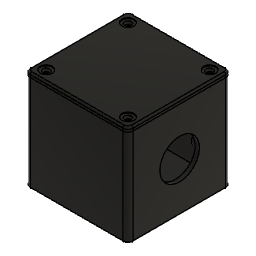
Transmitter_Box (Autodesk Fusion 360 design; units mm, degrees)
Autodesk Fusion 360 part; units mm, degrees
sketch "Sketch1" plane through (0, 0, 0) normal (0, 0, 1) x (1, 0, 0)
  line L0 (30, -30) -> (-30, -30)
  line L1 (-30, -30) -> (-30, 30)
  line L2 (-30, 30) -> (30, 30)
  line L3 (30, 30) -> (30, -30)
  line L4 (30, -30) -> (-30, 30) construction
  line L5 (-30, -30) -> (30, 30) construction
  dimension "d1" = 60
  dimension "d2" = 60
  constraint horizontal L0
  constraint perpendicular L0 L1
  constraint parallel L0 L2
  constraint parallel L1 L3
  constraint coincident L4 origin
  constraint coincident L5 origin
  measures "d1" distance of L1.end L2.end
  measures "d2" distance of L0.end L1.end
extrude "Extrude1" add sketch "Sketch1" along normal blind 2.4 makes body 1
sketch "Sketch2" plane through (0, 0, 2.4) normal (0, 0, 1) x (-1, 0, 0)
  line L0 (-30, -30) -> (30, -30)
  line L1 (30, -30) -> (30, 30)
  line L2 (30, 30) -> (-30, 30)
  line L3 (-30, 30) -> (-30, -30)
  line L4 (-27.6, -27.6) -> (27.6, -27.6)
  line L5 (27.6, -27.6) -> (27.6, 27.6)
  line L6 (27.6, 27.6) -> (-27.6, 27.6)
  line L7 (-27.6, 27.6) -> (-27.6, -27.6)
  line L8 (-27.6, -27.6) -> (27.6, 27.6) construction
  line L9 (27.6, -27.6) -> (-27.6, 27.6) construction
  dimension "d7" = 2.4
  dimension "d8" = 2.4
  constraint horizontal L4
  constraint perpendicular L4 L5
  constraint parallel L4 L6
  constraint parallel L5 L7
  constraint coincident L8 origin
  constraint coincident L9 origin
  measures "d7" distance of L0 L4
  measures "d8" distance of L1 L5
extrude "Extrude2" add sketch "Sketch2" along normal blind 54 bodies 1
sketch "Sketch3" plane through (0, 0, 56.4) normal (0, 0, 1) x (-1, 0, 0)
  line L0 (-27.6, -27.6) -> (-27.6, 27.6)
  line L1 (-27.6, 27.6) -> (27.6, 27.6)
  line L2 (27.6, 27.6) -> (27.6, -27.6)
  line L3 (27.6, -27.6) -> (-27.6, -27.6)
  line L4 (-30, 30) -> (-30, -30)
  line L5 (-30, -30) -> (30, -30)
  line L6 (30, -30) -> (30, 30)
  line L7 (30, 30) -> (-30, 30)
  line L8 (-30, 30) -> (30, 30)
  line L9 (30, 30) -> (30, -30)
  line L10 (30, -30) -> (-30, -30)
  line L11 (-30, -30) -> (-30, 30)
  constraint horizontal L8
  constraint vertical L9
  constraint horizontal L10
  constraint vertical L11
  constraint coincident L5.end L6.start
  constraint coincident L4.start L7.end
extrude "Extrude3" add sketch "Sketch3" along normal blind 2.4 separate body contours L0 L1 L2 L3 | L4 L5 L6 L7 L8 L9 L10 L11 makes body 2
sketch "Sketch4" plane through (-27.6, 0, 0) normal (1, 0, 0) x (0, 1, 0)
  line L0 (-27.6, 2.4) -> (27.6, 2.4)
  line L1 (27.6, 2.4) -> (27.6, 56.4)
  line L2 (27.6, 56.4) -> (-27.6, 56.4)
  line L3 (-27.6, 56.4) -> (-27.6, 2.4)
  line L4 (-27.6, 56.4) -> (-17.6, 56.4)
  line L5 (-17.6, 56.4) -> (-17.6, 52.4)
  line L6 (-17.6, 52.4) -> (-27.6, 52.4)
  line L7 (-27.6, 52.4) -> (-27.6, 56.4)
  line L8 (27.6, 56.4) -> (17.6, 56.4)
  line L9 (17.6, 56.4) -> (17.6, 52.4)
  line L10 (17.6, 52.4) -> (27.6, 52.4)
  line L11 (27.6, 52.4) -> (27.6, 56.4)
  dimension "d13" = 10
  dimension "d14" = 10
  dimension "d22" = 4
  dimension "d23" = 4
  constraint horizontal L4
  constraint vertical L5
  constraint horizontal L6
  constraint vertical L7
  constraint coincident L2.end L3.start
  constraint horizontal L8
  constraint vertical L9
  constraint horizontal L10
  constraint vertical L11
  constraint coincident L1.end L2.start
  measures "d13" distance of L5 L7
  measures "d14" distance of L9 L11
  measures "d22" distance of L4.end L5.end
  measures "d23" distance of L8.end L9.end
extrude "Extrude4" add sketch "Sketch4" along normal blind 10 contours L2 L3 L4 L5 L6 L7 | L1 L2 L8 L9 L10 L11 bodies 1
mirror "Mirror1" about plane through (0, 0, 0) normal (1, 0, 0) of "Extrude4"
sketch "Sketch8" plane through (0, 0, 56.4) normal (0, 0, 1) x (-1, 0, 0)
  line L0 (-27.6, -17.6) -> (-27.6, 17.6)
  line L1 (-27.6, 17.6) -> (-17.6, 17.6)
  line L2 (-17.6, 17.6) -> (-17.6, 27.6)
  line L3 (-17.6, 27.6) -> (17.6, 27.6)
  line L4 (17.6, 27.6) -> (17.6, 17.6)
  line L5 (17.6, 17.6) -> (27.6, 17.6)
  line L6 (27.6, 17.6) -> (27.6, -17.6)
  line L7 (27.6, -17.6) -> (17.6, -17.6)
  line L8 (17.6, -17.6) -> (17.6, -27.6)
  line L9 (17.6, -27.6) -> (-17.6, -27.6)
  line L10 (-17.6, -27.6) -> (-17.6, -17.6)
  line L11 (-17.6, -17.6) -> (-27.6, -17.6)
  line L12 (-30, 30) -> (-30, -30)
  line L13 (-30, -30) -> (30, -30)
  line L14 (30, -30) -> (30, 30)
  line L15 (30, 30) -> (-30, 30)
  circle A0 centre (-23.8, 23.8) radius 1.25
  circle A1 centre (23.8, 23.8) radius 1.25
  dimension "d27" = 2.5
  dimension "d28" = 6.2
  dimension "d29" = 6.2
  dimension "d30" = 2.5
  dimension "d31" = 6.2
  dimension "d32" = 6.2
  measures "d27" diameter of A0
  measures "d28" distance of L2 A0.centre
  measures "d29" distance of L1 A0.centre
  measures "d30" diameter of A1
  measures "d31" distance of L15 A1.centre
  measures "d32" distance of L14 A1.centre
extrude "Extrude5" cut sketch "Sketch8" against normal blind 4 contours A0 | A1 bodies 1
mirror "Mirror2" about plane through (0, 0, 0) normal (0, 1, 0) of "Extrude5"
sketch "Sketch9" plane through (0, 0, 58.8) normal (0, 0, 1) x (-1, 0, 0)
  line L0 (-30, -30) -> (30, -30)
  line L1 (30, -30) -> (30, 30)
  line L2 (30, 30) -> (-30, 30)
  line L3 (-30, 30) -> (-30, -30)
  circle A0 centre (-23.8, 23.8) radius 2
  circle A1 centre (23.8, 23.8) radius 2
  dimension "d37" = 4
  dimension "d38" = 6.2
  dimension "d39" = 6.2
  dimension "d40" = 4
  dimension "d41" = 6.2
  dimension "d42" = 6.2
  measures "d37" diameter of A0
  measures "d38" distance of L2 A0.centre
  measures "d39" distance of L3 A0.centre
  measures "d40" diameter of A1
  measures "d41" distance of L2 A1.centre
  measures "d42" distance of L1 A1.centre
extrude "Extrude6" cut sketch "Sketch9" against normal blind 2.4 contours A0 | A1 bodies 2
mirror "Mirror3" about plane through (0, 0, 0) normal (0, 1, 0) of "Extrude6"
sketch "Sketch10" plane through (0, 0, 58.8) normal (0, 0, 1) x (-1, 0, 0)
  circle A0 centre (-23.8, -23.8) radius 2
  circle A1 centre (23.8, -23.8) radius 2
  circle A2 centre (-23.8, 23.8) radius 2
  circle A3 centre (23.8, 23.8) radius 2
  line L0 (-30, -30) -> (30, -30)
  line L1 (30, -30) -> (30, 30)
  line L2 (30, 30) -> (-30, 30)
  line L3 (-30, 30) -> (-30, -30)
  circle A4 centre (-23.8, 23.8) radius 3.5
  circle A5 centre (-23.8, -23.8) radius 3.5
  dimension "d47" = 7
  dimension "d49" = 7
  constraint concentric A2 A4
  constraint concentric A0 A5
  measures "d47" diameter of A4
  measures "d49" diameter of A5
extrude "Extrude7" cut sketch "Sketch10" against normal blind 0.5 contours A4 | A5 bodies 2
mirror "Mirror4" about plane through (0, 0, 0) normal (1, 0, 0) of "Extrude7"
fillet "Fillet1" radius 5 4 edges at (-17.6, -17.6, 54.4) (-17.6, 17.6, 54.4) (17.6, 17.6, 54.4) (17.6, -17.6, 54.4) on bodies 1
fillet "Fillet2" radius 3 4 edges at (30, 30, 28.2) (30, -30, 28.2) (-30, -30, 28.2) (-30, 30, 28.2) on bodies 1
fillet "Fillet4" radius 3 4 edges at (30, 30, 57.6) (30, -30, 57.6) (-30, -30, 57.6) (-30, 30, 57.6) on bodies 2
sketch "Sketch12" plane through (0, 30, 0) normal (0, 1, 0) x (-1, 0, 0)
  line L0 (27, 0) -> (27, 56.4)
  line L1 (27, 56.4) -> (-27, 56.4)
  line L2 (-27, 56.4) -> (-27, 0)
  line L3 (-27, 0) -> (27, 0)
  line L4 (-3.75, 18.7) -> (3.75, 18.7)
  line L5 (3.75, 18.7) -> (3.75, 16.85)
  line L6 (3.75, 16.85) -> (3.25, 16.5)
  line L7 (3.25, 16.5) -> (3.25, 15)
  line L8 (3.25, 15) -> (-3.25, 15)
  line L9 (-3.25, 15) -> (-3.25, 16.5)
  line L10 (-3.25, 16.5) -> (-3.75, 16.85)
  line L11 (-3.75, 16.85) -> (-3.75, 18.7)
  constraint horizontal L4
  constraint perpendicular L4 L5
  constraint perpendicular L4 L7
  constraint perpendicular L7 L8
  constraint perpendicular L4 L9
  constraint perpendicular L4 L11
sketch "Sketch13" plane through (0, 27.6, 0) normal (0, 1, 0) x (-1, 0, 0)
  line L0 (27, 0) -> (27, 56.4)
  line L1 (27, 56.4) -> (-27, 56.4)
  line L2 (-27, 56.4) -> (-27, 0)
  line L3 (-27, 0) -> (27, 0)
  line L4 (3.75, 19.81) -> (-3.75, 19.81)
  line L5 (-3.75, 19.81) -> (-3.75, 17.96)
  line L6 (-3.75, 17.96) -> (-3.25, 17.61)
  line L7 (-3.25, 17.61) -> (-3.25, 16.11)
  line L8 (-3.25, 16.11) -> (3.25, 16.11)
  line L9 (3.25, 16.11) -> (3.25, 17.61)
  line L10 (3.25, 17.61) -> (3.75, 17.96)
  line L11 (3.75, 17.96) -> (3.75, 19.81)
  line L12 (-3.45, 19.51) -> (3.45, 19.51)
  line L13 (3.45, 19.51) -> (3.45, 18.1162)
  line L14 (3.45, 18.1162) -> (2.95, 17.7662)
  line L15 (2.95, 17.7662) -> (2.95, 16.41)
  line L16 (2.95, 16.41) -> (-2.95, 16.41)
  line L17 (-2.95, 16.41) -> (-2.95, 17.7662)
  line L18 (-2.95, 17.7662) -> (-3.45, 18.1162)
  line L19 (-3.45, 18.1162) -> (-3.45, 19.51)
  line L20 (-4.15, 17.7517) -> (-3.65, 17.4017)
  line L21 (-3.65, 17.4017) -> (-3.65, 15.71)
  line L22 (-3.65, 15.71) -> (3.65, 15.71)
  line L23 (3.65, 15.71) -> (3.65, 17.4017)
  line L24 (3.65, 17.4017) -> (4.15, 17.7517)
  line L25 (4.15, 17.7517) -> (4.15, 20.21)
  line L26 (4.15, 20.21) -> (-4.15, 20.21)
  line L27 (-4.15, 20.21) -> (-4.15, 17.7517)
  line L28 (8.95, 16.11) -> (-8.95, 16.11)
  line L29 (-8.95, 16.11) -> (-8.95, 14.51)
  line L30 (-8.95, 14.51) -> (8.95, 14.51)
  line L31 (8.95, 14.51) -> (8.95, 16.11)
  line L32 (-9.35, 14.11) -> (9.35, 14.11)
  line L33 (9.35, 14.11) -> (9.35, 16.51)
  line L34 (9.35, 16.51) -> (-9.35, 16.51)
  line L35 (-9.35, 16.51) -> (-9.35, 14.11)
  line L36 (-27.6, 52.4) -> (-17.6, 52.4)
  line L37 (-17.6, 52.4) -> (-17.6, 56.4)
  line L38 (-17.6, 56.4) -> (17.6, 56.4)
  line L39 (17.6, 56.4) -> (17.6, 52.4)
  line L40 (17.6, 52.4) -> (27.6, 52.4)
  line L41 (27.6, 52.4) -> (27.6, 2.4)
  line L42 (27.6, 2.4) -> (-27.6, 2.4)
  line L43 (-27.6, 2.4) -> (-27.6, 52.4)
  dimension "d79" = 0.4
  dimension "d80" = 0.4
extrude "Extrude10" cut sketch "Sketch13" along normal through all contours L4 L5 L6 L7 L9 L10 L11 L12 L13 L14 L15 L17 L18 L19 L34 | L4 L5 L6 L7 L9 L10 L11 L20 L21 L23 L24 L25 L26 L27 L34 | L9 L23 L28 L34 | L7 L8 L9 L15 L16 L17 L28 L34 | L7 L21 L28 L34 | L8 L21 L22 L23 L28 | L12 L13 L14 L15 L17 L18 L19 L34 | L15 L16 L17 L34 bodies 1
extrude "Extrude11" cut sketch "Sketch13" along normal blind 1 contours L9 L23 L28 L34 | L7 L8 L9 L15 L16 L17 L28 L34 | L7 L21 L28 L34 | L8 L21 L22 L23 L28 | L21 L23 L28 L29 L30 L31 L32 L33 L34 L35 | L15 L16 L17 L34 | L21 L22 L23 L28 L29 L30 L31 bodies 1
sketch "Sketch28" plane through (0, 27.6, 0) normal (0, -1, 0) x (1, 0, 0)
  line L0 (-9.35, 16.51) -> (-3.65, 16.51)
  line L1 (-3.65, 16.51) -> (-3.65, 17.4017)
  line L2 (-3.65, 17.4017) -> (-4.15, 17.7517)
  line L3 (-4.15, 17.7517) -> (-4.15, 20.21)
  line L4 (-4.15, 20.21) -> (4.15, 20.21)
  line L5 (4.15, 20.21) -> (4.15, 17.7517)
  line L6 (4.15, 17.7517) -> (3.65, 17.4017)
  line L7 (3.65, 17.4017) -> (3.65, 16.51)
  line L8 (3.65, 16.51) -> (9.35, 16.51)
  line L9 (9.35, 16.51) -> (9.35, 14.11)
  line L10 (9.35, 14.11) -> (-9.35, 14.11)
  line L11 (-9.35, 14.11) -> (-9.35, 16.51)
  line L12 (27.6, 52.4) -> (17.6, 52.4)
  line L13 (17.6, 52.4) -> (17.6, 56.4)
  line L14 (17.6, 56.4) -> (-17.6, 56.4)
  line L15 (-17.6, 56.4) -> (-17.6, 52.4)
  line L16 (-17.6, 52.4) -> (-27.6, 52.4)
  line L17 (-27.6, 52.4) -> (-27.6, 2.4)
  line L18 (-27.6, 2.4) -> (27.6, 2.4)
  line L19 (27.6, 2.4) -> (27.6, 52.4)
  line L20 (-4.0784, 37.8398) -> (4.0816, 37.8398)
  arc A0 (4.3816, 37.5398) -> (4.0816, 37.8398) centre (4.0816, 37.5398) ccw
  line L21 (4.3816, 37.5398) -> (4.3816, 27.2398)
  arc A1 (-4.0784, 37.8398) -> (-4.3784, 37.5398) centre (-4.0784, 37.5398) ccw
  line L22 (-4.3784, 27.2398) -> (-4.3784, 37.5398)
  line L23 (4.0816, 27.0398) -> (-4.0784, 27.0398)
  arc A2 (-4.3784, 27.2398) -> (-4.1784, 27.0398) centre (-4.1784, 27.2398) ccw
  line L24 (-4.0784, 27.0398) -> (-4.1784, 27.0398)
  arc A3 (4.1816, 27.0398) -> (4.3816, 27.2398) centre (4.1816, 27.2398) ccw
  line L25 (4.1816, 27.0398) -> (4.0816, 27.0398)
  circle A4 centre (0.0016, 33.3598) radius 3
  line L26 (4.1816, 26.6398) -> (4.0816, 26.6398)
  line L27 (4.0816, 26.6398) -> (-4.0784, 26.6398)
  line L28 (-4.0784, 26.6398) -> (-4.1784, 26.6398)
  arc A5 (-4.7784, 27.2398) -> (-4.1784, 26.6398) centre (-4.1784, 27.2398) ccw
  line L29 (-4.7784, 27.2398) -> (-4.7784, 37.5398)
  arc A6 (-4.0784, 38.2398) -> (-4.7784, 37.5398) centre (-4.0784, 37.5398) ccw
  line L30 (-4.0784, 38.2398) -> (4.0816, 38.2398)
  arc A7 (4.7816, 37.5398) -> (4.0816, 38.2398) centre (4.0816, 37.5398) ccw
  line L31 (4.7816, 37.5398) -> (4.7816, 27.2398)
  arc A8 (4.1816, 26.6398) -> (4.7816, 27.2398) centre (4.1816, 27.2398) ccw
  circle A9 centre (0.0016, 33.3598) radius 3.4
  dimension "d228" = -0.4
  dimension "d229" = 0.4
extrude "Extrude29" cut sketch "Sketch28" against normal through all contours A4 | A9 bodies 1
extrude "Extrude30" cut sketch "Sketch28" against normal blind 1.2 contours L20 A0 L21 A1 L22 L23 A2 L24 A3 L25 | L26 L27 L28 A5 L29 A6 L30 A7 L31 A8 bodies 1
fillet "Fillet13" radius 1 16 edges at (29.1213, -29.1213, 0) (30, 0, 0) (29.1213, 29.1213, 0) (0, 30, 0) (-29.1213, 29.1213, 0) (-30, 0, 0) (-29.1213, -29.1213, 0) (0, -30, 0) (29.1213, 29.1213, 58.8) (0, 30, 58.8) (-29.1213, 29.1213, 58.8) (-30, 0, 58.8) (-29.1213, -29.1213, 58.8) (0, -30, 58.8) (29.1213, -29.1213, 58.8) (30, 0, 58.8) on bodies 1 2
sketch "Sketch30" plane through (0, -30, 0) normal (0, -1, 0) x (1, 0, 0)
  line L0 (-27, 1) -> (27, 1)
  line L1 (27, 1) -> (27, 56.4)
  line L2 (27, 56.4) -> (-27, 56.4)
  line L3 (-27, 56.4) -> (-27, 1)
  line L4 (-15.923, 16.6996) -> (-15.923, 40.6996)
  line L5 (-15.923, 40.6996) -> (16.077, 40.6996)
  line L6 (16.077, 40.6996) -> (16.077, 16.6996)
  line L7 (16.077, 16.6996) -> (-15.923, 16.6996)
  arc A0 (0.077, 40.1996) -> (-11.423, 28.6996) centre (0.077, 28.6996) ccw
  arc A1 (11.577, 28.6996) -> (0.077, 40.1996) centre (0.077, 28.6996) ccw
  arc A2 (0.077, 17.1996) -> (11.577, 28.6996) centre (0.077, 28.6996) ccw
  arc A3 (-11.423, 28.6996) -> (0.077, 17.1996) centre (0.077, 28.6996) ccw
  arc A4 (-14.423, 27.6996) -> (-14.423, 29.6996) centre (-14.423, 28.6996) ccw
  arc A5 (-14.423, 29.6996) -> (-14.423, 27.6996) centre (-14.423, 28.6996) ccw
  arc A6 (14.577, 29.6996) -> (14.577, 27.6996) centre (14.577, 28.6996) ccw
  arc A7 (14.577, 27.6996) -> (14.577, 29.6996) centre (14.577, 28.6996) ccw
  arc A8 (-14.423, 26.4496) -> (-14.423, 30.9496) centre (-14.423, 28.6996) ccw
  arc A9 (-14.423, 30.9496) -> (-14.423, 26.4496) centre (-14.423, 28.6996) ccw
  line L8 (-8.923, 40.6996) -> (9.077, 40.6996)
  arc A10 (-8.923, 40.6996) -> (-11.923, 37.6996) centre (-8.923, 37.6996) ccw
  line L9 (-11.923, 19.6996) -> (-11.923, 37.6996)
  arc A11 (-11.923, 19.6996) -> (-8.923, 16.6996) centre (-8.923, 19.6996) ccw
  arc A12 (12.077, 37.6996) -> (9.077, 40.6996) centre (9.077, 37.6996) ccw
  line L10 (12.077, 37.6996) -> (12.077, 19.6996)
  arc A13 (9.077, 16.6996) -> (12.077, 19.6996) centre (9.077, 19.6996) ccw
  line L11 (9.077, 16.6996) -> (-8.923, 16.6996)
  arc A14 (14.577, 26.4496) -> (14.577, 30.9496) centre (14.577, 28.6996) ccw
  arc A15 (14.577, 30.9496) -> (14.577, 26.4496) centre (14.577, 28.6996) ccw
  dimension "d237" = 1.25
  dimension "d238" = 1.25
extrude "Extrude31" cut sketch "Sketch30" against normal blind 2.4 contours A0 A1 A2 A3 bodies 1
extrude "Extrude32" add sketch "Sketch30" against normal blind 5.5 contours L4 A9 | L4 A8 A9 | L6 A14 A15 | L6 A14 bodies 1
sketch "Sketch31" plane through (0, 30, 0) normal (0, 1, 0) x (-1, 0, 0)
  line L0 (-27, 1) -> (27, 1)
  line L1 (27, 1) -> (27, 56.4)
  line L2 (27, 56.4) -> (-27, 56.4)
  line L3 (-27, 56.4) -> (-27, 1)
  circle A0 centre (-0.0016, 33.3598) radius 3.4
  line L4 (3.65, 15.71) -> (-3.65, 15.71)
  line L5 (-3.65, 15.71) -> (-3.65, 17.4017)
  line L6 (-3.65, 17.4017) -> (-4.15, 17.7517)
  line L7 (-4.15, 17.7517) -> (-4.15, 20.21)
  line L8 (-4.15, 20.21) -> (4.15, 20.21)
  line L9 (4.15, 20.21) -> (4.15, 17.7517)
  line L10 (4.15, 17.7517) -> (3.65, 17.4017)
  line L11 (3.65, 17.4017) -> (3.65, 15.71)
  circle A1 centre (0, 47.5) radius 2.9
  circle A2 centre (0, 47.5) radius 3.1
  dimension "d241" = 0.2
extrude "Extrude33" cut sketch "Sketch31" against normal blind 2.4 contours A1 | A2 bodies 1
move_body "Move1" bodies 1 2 to x (0, 1, 0) y (-1, 0, 0) z (0, 0, 1) at (0, 0, 0)
equation "d3 = boxWidth"
equation "d7 = boxWidth"
equation "d8 = boxWidth"
equation "d11 = boxWidth"
equation "boxWidth = 2.4 mm"
equation "d23 = d22"
equation "d27 = boxScrewHoleWidth"
equation "d30 = boxScrewHoleWidth"
equation "d43 = -boxWidth"
equation "d47 = boxSanfren"
equation "boxSanfren = 7 mm"
equation "d49 = boxSanfren"
equation "boxSanfrenDepth = 0.5 mm"
equation "d51 = -boxSanfrenDepth"
equation "boxScrewHoleWidth = 2.5 mm"
equation "d163 = 1 mm"
equation "d176 = d163"
equation "d177 = 6 mm"
equation "d180 = d177"
equation "d181 = d176"
named bodies: "Case", "Cap"
